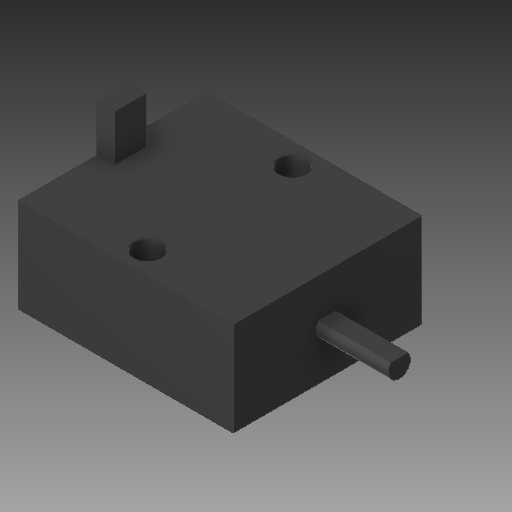
# Autodesk Inventor part: MotorWithEnclosure
Saved by Autodesk Inventor 2018 (Build 220112000, 112)
## iProperties
Created: 2018-01-17
Part Number: MotorWithEnclosure
Material: ABS Plastic
Document SubType Name: Modeling
Designer: mmarkle
Density: 1.06 g/cm^3
Appearance: Smooth - Black
Mass: 9.72914 g
Surface Area: 32.8446 cm^2
Volume: 9.17844 cm^3
Author: mmarkle
Autodesk Inventor part; units mm, degrees
ref_plane "YZ Plane" through (0, 0, 0) normal (1, 0, 0) x (0, 1, 0)
ref_plane "XZ Plane" through (0, 0, 0) normal (0, 1, 0) x (-1, 0, 0)
ref_plane "XY Plane" through (0, 0, 0) normal (0, 0, 1) x (1, 0, 0)
sketch "Sketch1" plane through (0, 0, 0) normal (0, 1, 0) x (-1, 0, 0)
  line L0 (-14.478, 12.7) -> (14.478, 12.7)
  line L1 (14.478, 12.7) -> (14.478, -12.7)
  line L2 (14.478, -12.7) -> (-14.478, -12.7)
  line L3 (-14.478, -12.7) -> (-14.478, 12.7)
  line L4 (-14.478, 12.7) -> (14.478, -12.7) construction
  line L5 (14.478, 12.7) -> (-14.478, -12.7) construction
  point P0 (0, 0)
  dimension "d0" = 28.956
  dimension "d1" = 25.4
  constraints: 12 end point, 2 midpoint, 2 parallel, 1 horizontal, 1 perpendicular
  measures "d0" distance of L1.end L2.end
  measures "d1" distance of L0.end L1.end
extrude "Extrusion1" add sketch "Sketch1" along normal blind 12.7
sketch "Sketch2" plane through (0, 12.7, 0) normal (0, 1, 0) x (1, 0, 0)
  point P0 (0, 0)
  point P1 (0, -9.779)
  point P2 (0, 9.779)
  dimension "d4" = 9.779
  dimension "d5" = 19.558
  measures "d4" distance of point (0, -9.779) point (0, 0)
  measures "d5" distance of point (0, -9.779) point (0, 9.779)
hole "Hole1" at (0, 12.7, 9.779) at (0, 12.7, -9.779) direction (0, -1, 0) diameter 3.81 end through all clearance for "Flat Head Machine Screw (82)" size "#6" standard "Ansi Unified Screw Threads"
sketch "Sketch3" plane through (14.478, 0, 12.7) normal (1, 0, 0) x (0, 0, -1)
  circle A0 centre (12.7, 6.35) radius 1.5
  line L0 (25.4, 0) -> (0, 0) projected
  line L1 (0, 12.7) -> (25.4, 12.7) projected
  line L2 (11.582, 7.35) -> (13.818, 7.35)
  point P0 (12.7, 0)
  point P1 (12.7, 0)
  dimension "d13" = 3
  dimension "d14" = 6.35
  dimension "d15" = 12.7
  dimension "d18" = 1
  constraints: 2 end point, 2 point on circle, 1 centre point, 1 horizontal, 1 midpoint, 1 vertical alignment
  measures "d13" diameter of A0
  measures "d14" distance of point (12.7, 0) A0.centre
  measures "d15" distance from line of L1 point (12.7, 0)
  measures "d18" distance from line of A0.centre L2
extrude "Extrusion3" add sketch "Sketch3" along normal blind 9.7 contours A0 L2 picked at (12.7594, 6.5202)
sketch "Sketch4" plane through (0, 12.7, 0) normal (0, 1, 0) x (1, 0, 0)
  line L0 (-14.478, -2.1797) -> (-12.0814, -2.1797)
  line L1 (-12.0814, -2.1797) -> (-12.0814, 2.1797)
  line L2 (-12.0814, 2.1797) -> (-14.478, 2.1797)
  line L3 (-14.478, 2.1797) -> (-14.478, -2.1797)
  line L4 (-14.478, -2.1797) -> (-12.0814, 2.1797) construction
  line L5 (-12.0814, -2.1797) -> (-14.478, 2.1797) construction
  line L6 (-14.478, 12.7) -> (-14.478, -12.7) projected
  point P0 (0, 0)
  point P1 (-13.2797, 0)
  point P2 (-13.2797, 0)
  constraints: 12 end point, 3 midpoint, 2 parallel, 1 collinear, 1 horizontal, 1 horizontal alignment, 1 perpendicular
extrude "Extrusion4" add sketch "Sketch4" along normal blind 6.35
equation "\"d14\" = 0.5 * d15"
body "Solid1"
